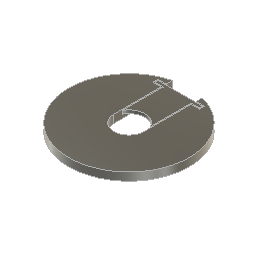
cap v4 (Autodesk Fusion 360 design; units mm, degrees)
Autodesk Fusion 360 part; units mm, degrees
note: some values were not read from the file. Set by a fixed rule: which sketch regions a step uses.
sketch "Sketch1" plane through (0, 0, 0) normal (0, 0, 1) x (1, 0, 0)
  circle A0 centre (0, 0) radius 30
  circle A1 centre (0, 0) radius 7.5
  line L0 (-7.5, 0) -> (-7.5, 29.0474)
  line L1 (7.5, 0) -> (7.5, 29.0474)
  dimension "d1" = 60
  dimension "d2" = 15
  constraint coincident A0.centre A1.centre
  constraint concentric A0 A1
  constraint coincident A1 L0.start
  constraint coincident A0 L0.end
  constraint tangent A1 L0
  constraint vertical L0
  constraint coincident A1 L1.start
  constraint coincident A0 L1.end
  constraint tangent A1 L1
  constraint parallel L0 L1
  measures "d1" diameter of A0
  measures "d2" diameter of A1
extrude "Extrude1" add sketch "Sketch1" along normal blind 4 contours A0 A1 L0 L1 picked at (-22.4151, 1.0871) makes body 1
copy_body "Body->Comp1" bodies 1 removing the originals makes body 2 in component "cap"
sketch "Sketch2" plane through (0, 0, 4) normal (0, 0, 1) x (-1, 0, 0)
  line L0 (7.5, 0) -> (7.5, -29.0474)
  arc A0 (7.5, -29.0474) -> (-7.5, -29.0474) centre (0, 0) ccw
  line L1 (-7.5, -29.0474) -> (-7.5, 0)
  arc A1 (7.5, 0) -> (-7.5, 0) centre (0, 0) ccw
  line L2 (7.5, -25.9986) -> (11.5, -25.9986)
  line L3 (11.5, -25.9986) -> (11.5, -23.4986)
  line L4 (11.5, -23.4986) -> (7.5, -23.4986)
  line L5 (7.5, -23.4986) -> (7.5, -25.9986)
  line L6 (0, -31.0207) -> (0, -18.5293)
  line L7 (-7.5, -25.9986) -> (-11.5, -25.9986)
  line L8 (-11.5, -25.9986) -> (-11.5, -23.4986)
  line L9 (-11.5, -23.4986) -> (-7.5, -23.4986)
  line L10 (-7.5, -23.4986) -> (-7.5, -25.9986)
  dimension "d5" = 4
  dimension "d6" = 2.5
  constraint horizontal L2
  constraint vertical L3
  constraint horizontal L4
  constraint vertical L5
  constraint coincident L0 L2.start
  constraint vertical L6
  constraint symmetric L2.start L6 L7.start
  constraint symmetric L2.end L6 L7.end
  constraint symmetric L3.end L6 L8.end
  constraint symmetric L4.end L6 L9.end
  measures "d5" distance of L2.start L2.end
  measures "d6" distance of L2.start L4.end
extrude "Extrude1'" cut sketch "Sketch2" against normal blind 2 contours L0 L2 L3 L4 L5 | L1 L7 L8 L9 L10 bodies 2 in component "cap"
sketch "Sketch3" plane through (0, 0, 4) normal (0, 0, 1) x (-1, 0, 0)
  line L0 (11.5, -25.9986) -> (7.5, -25.9986)
  line L1 (7.5, -25.9986) -> (7.5, -29.0474)
  arc A0 (7.5, -29.0474) -> (-7.5, -29.0474) centre (0, 0) ccw
  line L2 (-7.5, -29.0474) -> (-7.5, -25.9986)
  line L3 (-7.5, -25.9986) -> (-11.5, -25.9986)
  line L4 (-11.5, -25.9986) -> (-11.5, -23.4986)
  line L5 (-11.5, -23.4986) -> (-7.5, -23.4986)
  line L6 (-7.5, -23.4986) -> (-7.5, 0)
  arc A1 (7.5, 0) -> (-7.5, 0) centre (0, 0) ccw
  line L7 (7.5, 0) -> (7.5, -23.4986)
  line L8 (7.5, -23.4986) -> (11.5, -23.4986)
  line L9 (11.5, -23.4986) -> (11.5, -25.9986)
  circle A2 centre (0, 0) radius 7.5
  line L10 (7.5, 0) -> (7.5, -23.4986)
  line L11 (7.5, -25.9986) -> (-7.5, -25.9986)
  line L12 (7.5, -25.9986) -> (11.5, -25.9986)
  line L13 (11.5, -23.4986) -> (7.5, -23.4986)
  line L14 (-7.5, -25.9986) -> (-11.5, -25.9986)
  line L15 (-11.5, -23.4986) -> (-7.5, -23.4986)
  line L16 (-7.5, 0) -> (-7.5, -23.4986)
  line L17 (11.5, -23.4986) -> (11.5, -25.9986)
  line L18 (-11.5, -23.4986) -> (-11.5, -25.9986)
  circle A3 centre (0, 0) radius 7.9
  line L19 (7, 0) -> (7, -23.9986)
  line L20 (11, -23.9986) -> (7, -23.9986)
  line L21 (11, -23.9986) -> (11, -25.4986)
  line L22 (7.5, -25.4986) -> (11, -25.4986)
  line L23 (7.5, -25.4986) -> (-7.5, -25.4986)
  line L24 (-7.5, -25.4986) -> (-11, -25.4986)
  line L25 (-11, -23.9986) -> (-11, -25.4986)
  line L26 (-11, -23.9986) -> (-7, -23.9986)
  line L27 (-7, 0) -> (-7, -23.9986)
  dimension "d9" = 15
  dimension "d10" = 0.4
  dimension "d11" = -0.5
  constraint concentric A0 A2
  constraint coincident A1.start L7.start
  constraint coincident L7.end L8.start
  constraint coincident L0.end L1.start
  constraint coincident L2.end L3.start
  constraint coincident L0.start L9.end
  constraint coincident L8.end L9.start
  constraint coincident L3.end L4.start
  constraint coincident L4.end L5.start
  constraint coincident L5.end L6.start
  constraint coincident L6.end A1.end
  measures "d9" diameter of A2
extrude "Extrude1''" add sketch "Sketch3" against normal blind 1.6 separate body contours A3 L19 L20 L21 L22 L23 L24 L25 L26 L27 makes body 3 in component "cover"
component "cap" placed x (1, 0, 0) y (0, 1, 0) z (0, 0, 1) at (0, 0, 0)
component "cover" placed x (1, 0, 0) y (0, 1, 0) z (0, 0, 1) at (0, 0, 0)
